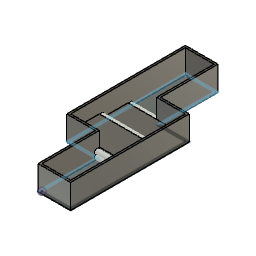
Hurdles v1 (Autodesk Fusion 360 design; units mm, degrees)
Autodesk Fusion 360 part; units mm, degrees
sketch "Sketch1" plane through (0, 0, 0) normal (0, 0, 1) x (1, 0, 0)
  line L0 (0, 0) -> (300, 0)
  line L1 (300, 0) -> (300, 1200)
  line L2 (300, 1200) -> (0, 1200)
  line L3 (0, 600) -> (-300, 600)
  line L4 (-300, 600) -> (-300, 1800)
  line L5 (-300, 1800) -> (0, 1800)
  line L6 (0, 1800) -> (0, 1200)
  line L7 (0, 0) -> (0, 600)
  line L8 (20, 1820) -> (20, 1220)
  line L9 (320, 1220) -> (20, 1220)
  line L10 (320, -20) -> (320, 1220)
  line L11 (-20, -20) -> (320, -20)
  line L12 (-20, -20) -> (-20, 580)
  line L13 (-20, 580) -> (-320, 580)
  line L14 (-320, 580) -> (-320, 1820)
  line L15 (-320, 1820) -> (20, 1820)
  dimension "d1" = 300
  dimension "d2" = 1200
  dimension "d3" = 300
  dimension "d4" = 1200
  dimension "d5" = -20
  constraint horizontal L0
  constraint vertical L1
  constraint horizontal L2
  constraint coincident L0.start L7.start
  constraint perpendicular L3 L4
  constraint perpendicular L4 L5
  constraint perpendicular L2 L6
  constraint perpendicular L3 L7
  measures "d1" distance of L0.start L0.end
  measures "d2" distance of L0.end L1.end
  measures "d3" distance of L3.start L3.end
  measures "d4" distance of L3.end L4.end
extrude "Extrude1" add sketch "Sketch1" along normal blind 400 makes body 1
extrude "Extrude2" add sketch "Sketch1" against normal blind 5 separate body contours L0 L1 L2 L3 L4 L5 L6 L7 makes body 2
extrude "Extrude3" add sketch "Sketch1" against normal blind 5 bodies 1 2
extrude "Extrude4" cut 1 faces at (-313.3333, 1400, 400) along direction (0, 0, -1) blind 100 on bodies 1 bodies 1
extrude "Extrude5" cut 1 faces at (-313.3333, 1400, 300) along direction (0, 0, -1) blind 50 on bodies 1 bodies 1
sketch "Sketch2" plane through (0, 0, 0) normal (1, 0, 0) x (0, 1, 0)
  line L0 (600, 250) -> (0, 250)
  line L1 (0, 250) -> (0, 0)
  line L2 (0, 0) -> (600, 0)
  line L3 (600, 0) -> (600, 250)
  line L4 (600, 0) -> (575, 0) construction
  line L5 (575, 0) -> (575, 25) construction
  circle A0 centre (575, 25) radius 25
  line L6 (575, 25) -> (575, 75) construction
  circle A1 centre (575, 75) radius 25
  dimension "d16" = 25
  dimension "d17" = 25
  dimension "d18" = 50
  dimension "d19" = 50
  dimension "d20" = 50
  constraint coincident L2.end L3.start
  constraint perpendicular L3 L4
  constraint perpendicular L4 L5
  constraint coincident L5.end A0.centre
  constraint parallel L5 L6
  constraint coincident L6.end A1.centre
  measures "d16" distance of L2.end L4.end
  measures "d17" distance of L4.end L5.end
  measures "d18" diameter of A0
  measures "d19" distance of L5.end L6.end
  measures "d20" diameter of A1
extrude "Extrude6" add sketch "Sketch2" along normal blind 300 separate body contours A1 | A0 makes body 3
box "BoxPrimitive1" add length 300 width 388.5404 height 100 placed x (0, 1, 0) y (-1, 0, 0) z (0, 0, 1) at (88.593, 600.0573, 0) bodies 1
extrude "Extrude7" add 1 faces at (88.593, 800.0573, 33.3333) along direction (1, 0, 0) blind 211.407 on bodies 1 bodies 1
sketch "Sketch4" plane through (-300, 0, 0) normal (1, 0, 0) x (0, 1, 0)
  line L0 (1800, 250) -> (600, 250)
  line L1 (600, 250) -> (600, 0)
  line L2 (600, 0) -> (1800, 0)
  line L3 (1800, 0) -> (1800, 250)
  line L4 (899.8838, 99.9399) -> (924.8838, 99.9399)
  line L5 (924.8838, 99.9399) -> (924.8838, 74.9399)
  circle A0 centre (924.8838, 74.9399) radius 25
  dimension "d30" = 25
  dimension "d31" = 25
  dimension "d32" = 50
  constraint horizontal L4
  constraint perpendicular L4 L5
  constraint coincident L5.end A0.centre
  measures "d30" distance of L4.start L4.end
  measures "d31" distance of L4.end L5.end
  measures "d32" diameter of A0
extrude "Extrude8" add sketch "Sketch4" along normal blind 600 separate body contours A0 makes body 4
sketch "Sketch5" plane through (0, 900.0573, 0) normal (0, 1, 0) x (-1, 0, 0)
  line L0 (-300, 0) -> (299.9474, 0)
  line L1 (299.9474, 0) -> (299.9474, 100)
  line L2 (299.9474, 100) -> (-300, 100)
  line L3 (-300, 100) -> (-300, 0)
  line L4 (-300, 0) -> (-300, 50) construction
  line L5 (-300, 50) -> (299.9474, 50)
  dimension "d35" = 50
  constraint coincident L0.start L3.end
  constraint perpendicular L0 L4
  constraint coincident L1 L5.end
  constraint perpendicular L1 L5
  measures "d35" distance of L0.start L4.end
extrude "Extrude9" add sketch "Sketch5" along normal blind 299.943 separate body contours L0 L1 L3 L5 makes body 5
sketch "Sketch6" plane through (0, 0, 0) normal (-1, 0, 0) x (0, -1, 0)
  line L0 (-1200, 250) -> (-1800, 250)
  line L1 (-1800, 250) -> (-1800, 0)
  line L2 (-1800, 0) -> (-1200, 0)
  line L3 (-1200, 0) -> (-1200, 250)
  line L4 (-1200, 0) -> (-1225, 0) construction
  line L5 (-1225, 0) -> (-1225, 25) construction
  circle A0 centre (-1225, 25) radius 25
  dimension "d38" = 25
  dimension "d39" = 25
  dimension "d40" = 50
  constraint coincident L2.end L3.start
  constraint perpendicular L3 L4
  constraint perpendicular L2 L5
  constraint coincident L5.end A0.centre
  measures "d38" distance of L2.end L4.end
  measures "d39" distance of L4.end L5.end
  measures "d40" diameter of A0
extrude "Extrude10" add sketch "Sketch6" along normal blind 300 separate body contours A0 makes body 6
